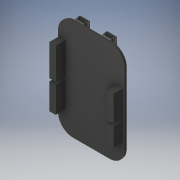
# Autodesk Inventor part: FRDM-KL25Z
Saved by Autodesk Inventor 2019 (Build 230136000, 136)
## iProperties
Created: 2019-07-30
Part Number: FRDM-KL25Z
Material: Résine phénolique
Document SubType Name: Modeling
Designer: Sébastien DI MERCURIO
Mass: 9.77702 g
Surface Area: 92.912 cm^2
Volume: 7.0848 cm^3
Density: 1.38 g/cm^3
Appearance: Lisse - Noir
Author: Sébastien DI MERCURIO
Autodesk Inventor part; units mm, degrees
ref_plane "YZ Plane" through (0, 0, 0) normal (1, 0, 0) x (0, 1, 0)
ref_plane "XZ Plane" through (0, 0, 0) normal (0, 1, 0) x (-1, 0, 0)
ref_plane "XY Plane" through (0, 0, 0) normal (0, 0, 1) x (1, 0, 0)
sketch "Esquisse1" plane through (0, 0, 0) normal (0, 0, 1) x (1, 0, 0)
  line L0 (0, 0) -> (54, 0)
  line L1 (54, 0) -> (54, 82)
  line L2 (54, 82) -> (0, 82)
  line L3 (0, 82) -> (0, 0)
  dimension "d0" = 54
  dimension "d1" = 82
  constraints: 8 end point, 2 parallel, 1 horizontal, 1 perpendicular
  measures "d0" distance between parallel lines of L1 L3
  measures "d1" distance between parallel lines of L0 L2
extrude "Extrusion1" add sketch "Esquisse1" along normal blind 1.6
fillet "Congé1" radius 12 4 edges at (0, 82, 0.8) (54, 82, 0.8) (54, 0, 0.8) (0, 0, 0.8)
sketch "Esquisse2" plane through (0, 0, 1.6) normal (0, 0, 1) x (1, 0, 0)
  line L0 (12, 0) -> (42, 0) projected
  line L1 (1, 65.8) -> (6, 65.8)
  line L2 (6, 65.8) -> (6, 40.3)
  line L3 (6, 40.3) -> (1, 40.3)
  line L4 (1, 40.3) -> (1, 65.8)
  line L5 (1, 38) -> (6, 38)
  line L6 (6, 38) -> (6, 17)
  line L7 (6, 17) -> (1, 17)
  line L8 (1, 17) -> (1, 38)
  line L9 (48, 32) -> (53, 32)
  line L10 (53, 32) -> (53, 17)
  line L11 (53, 17) -> (48, 17)
  line L12 (48, 17) -> (48, 32)
  line L13 (48, 55.3) -> (53, 55.3)
  line L14 (53, 55.3) -> (53, 34.3)
  line L15 (53, 34.3) -> (48, 34.3)
  line L16 (48, 34.3) -> (48, 55.3)
  line L17 (0, 70) -> (0, 12) projected
  line L18 (54, 12) -> (54, 70) projected
  point P0 (0, 0)
  dimension "d11" = 5
  dimension "d12" = 17
  dimension "d13" = 2.3
  dimension "d14" = 2.3
  dimension "d15" = 15
  dimension "d16" = 21
  dimension "d17" = 25.5
  dimension "d18" = 1
  dimension "d19" = 1
  constraints: 32 end point, 11 parallel, 4 horizontal, 4 perpendicular, 3 point on line, 1 collinear
  measures "d11" distance of L13.start L13.end
  measures "d12" distance between parallel lines of L0 L11
  measures "d13" distance between parallel lines of L9 L15
  measures "d14" distance between parallel lines of L5 L3
  measures "d15" distance of L9.end L10.end
  measures "d16" distance of L13.end L14.end
  measures "d17" distance of L3.end L1.start
  measures "d18" distance from line of L17 L7.end
  measures "d19" distance from line of L18 L10.end
extrude "Extrusion2" add sketch "Esquisse2" along normal blind 8
sketch "Esquisse3" plane through (0, 0, 0) normal (0, 0, -1) x (-1, 0, 0)
  line L0 (-12, 83) -> (-20, 83)
  line L1 (-20, 83) -> (-20, 73.5)
  line L2 (-20, 73.5) -> (-12, 73.5)
  line L3 (-12, 73.5) -> (-12, 83)
  line L4 (-34, 83) -> (-42, 83)
  line L5 (-42, 83) -> (-42, 73.5)
  line L6 (-42, 73.5) -> (-34, 73.5)
  line L7 (-34, 73.5) -> (-34, 83)
  line L8 (-42, 82) -> (-12, 82) projected
  line L9 (0, 70) -> (0, 12) projected
  line L10 (-54, 12) -> (-54, 70) projected
  point P0 (0, 0)
  dimension "d22" = 8
  dimension "d23" = 9.5
  dimension "d24" = 1
  dimension "d25" = 12
  dimension "d26" = 12
  constraints: 16 end point, 4 parallel, 2 horizontal, 2 perpendicular, 2 point on line, 1 collinear
  measures "d22" distance between parallel lines of L1 L3
  measures "d23" distance of L2.end L0.start
  measures "d24" distance between parallel lines of L8 L0
  measures "d25" distance between parallel lines of L9 L3
  measures "d26" distance between parallel lines of L10 L5
extrude "Extrusion3" add sketch "Esquisse3" along normal blind 4.2
sketch "Esquisse4" plane through (12, 83, 0) normal (0, 1, 0) x (1, 0, 0)
  line L0 (0, 0) -> (0.5, 0)
  line L1 (0.5, 0) -> (0.5, 2)
  line L2 (0.5, 2) -> (0, 2)
  line L3 (0, 2) -> (0, 0)
  line L4 (8, 0) -> (7.5, 0)
  line L5 (7.5, 0) -> (7.5, 2)
  line L6 (7.5, 2) -> (8, 2)
  line L7 (8, 2) -> (8, 0)
  line L8 (8, 0) -> (8, 4.2) projected
  line L9 (22, 0) -> (22, 4.2) projected
  line L10 (22, 0) -> (22.5, 0)
  line L11 (22.5, 0) -> (22.5, 2)
  line L12 (22.5, 2) -> (22, 2)
  line L13 (22, 2) -> (22, 0)
  line L14 (30, 0) -> (30, 4.2) projected
  line L15 (30, 0) -> (29.5, 0)
  line L16 (29.5, 0) -> (29.5, 2)
  line L17 (29.5, 2) -> (30, 2)
  line L18 (30, 2) -> (30, 0)
  line L19 (0, 0) -> (8, 0) projected
  line L20 (0, 0) -> (0, 4.2) projected
  point P0 (-12, 0)
  dimension "d29" = 0.5
  dimension "d30" = 2
  constraints: 32 end point, 8 parallel, 4 equal length, 4 horizontal, 4 perpendicular, 3 collinear, 3 point on line
  measures "d29" distance of L1.end L2.end
  measures "d30" distance from line of L0.start L2
extrude "Extrusion4" cut sketch "Esquisse4" against normal blind 2.2
fillet "Congé2" radius 0.25 8 edges at (34.5, 81.9, -2) (34, 81.9, -2) (41.5, 81.9, -2) (42, 81.9, -2) (19.5, 81.9, -2) (20, 81.9, -2) (12.5, 81.9, -2) (12, 81.9, -2)
shell "Coque1" thickness 0.6 removed faces 2 at (17.1749, 83, -3.4195) at (39.1749, 83, -3.4195)
equation "\"d14\" = d13"
equation "\"d19\" = d18"
equation "\"d26\" = d25"
